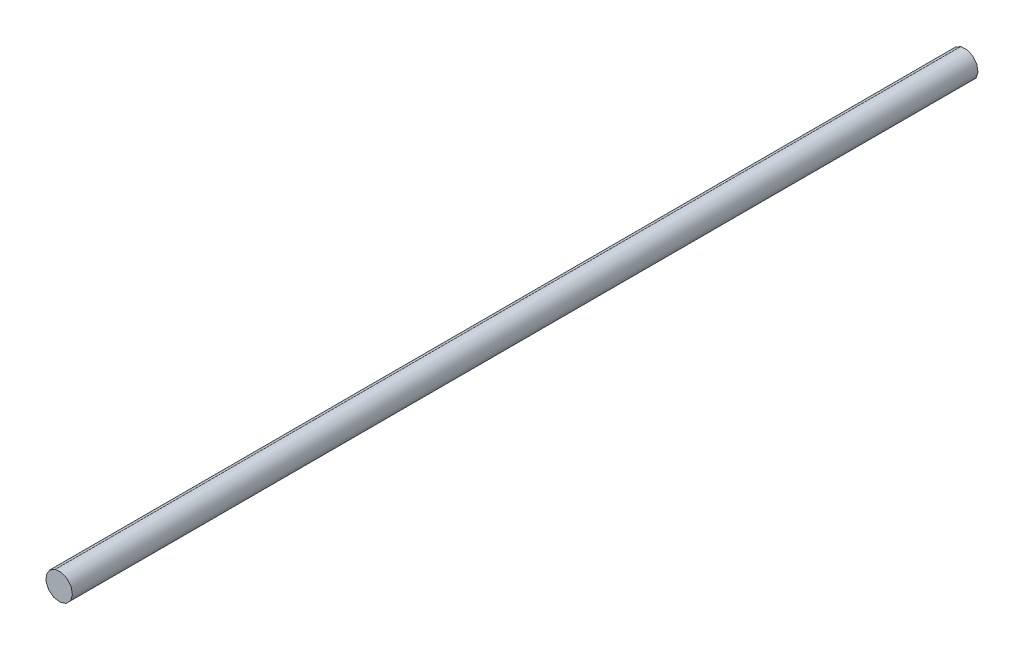
# Autodesk Inventor part: guida__Z
Saved by Autodesk Inventor 2014 SP1 (Build 180222100, 222)
## iProperties
Created: 2015-04-15
Part Number: guida__Z
Material: Generic
Document SubType Name: Modeling
Designer: Giorgio Nuzzo
Density: 1 g/cm^3
Appearance: Default
Author: Giorgio Nuzzo
Autodesk Inventor part; units mm, degrees
ref_plane "YZ Plane" through (0, 0, 0) normal (1, 0, 0) x (0, 1, 0)
ref_plane "XZ Plane" through (0, 0, 0) normal (0, 1, 0) x (-1, 0, 0)
ref_plane "Work Plane1" through (-6.5765, 0, 5) normal (0, 0, 1) x (-0.9529, 0.3031, 0)
sketch "Sketch1" plane through (-6.5765, 0, 5) normal (0, 0, 1) x (-0.9529, 0.3031, 0)
  circle A0 centre (0, 0) radius 5 projected
  point P0 (-6.2671, -1.9935)
ref_plane "Work Plane2" through (-15.5765, -8.1, -335) normal (0, 0, 1) x (1, 0, 0)
extrude "Extrusion1" add sketch "Sketch1" against normal up to surface (340 mm away)
body "Solid1"
